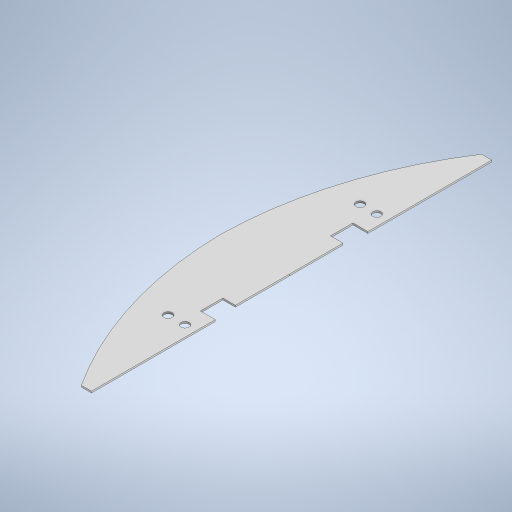
# Autodesk Inventor part: sensor3
Saved by Autodesk Inventor 2023 (Build 270158000, 158)
## iProperties
Created: 2023-08-10
Part Number: sensor3
Material: Genérico
Document SubType Name: Modeling
Designer: azeve
Density: 1 g/cm^3
Appearance: Padrão
Author: azeve
Autodesk Inventor part; units mm, degrees
ref_plane "YZ Plane" through (0, 0, 0) normal (1, 0, 0) x (0, 1, 0)
ref_plane "XZ Plane" through (0, 0, 0) normal (0, 1, 0) x (-1, 0, 0)
ref_plane "XY Plane" through (0, 0, 0) normal (0, 0, 1) x (1, 0, 0)
sketch "Esboço1" plane through (0, 0, 0) normal (0, 1, 0) x (-1, 0, 0)
  line L0 (-21.2717, 119.5968) -> (-21.2717, 45.5844)
  line L1 (-19.833, 32.1612) -> (-19.845, 0)
  line L2 (-19.845, 0) -> (21.2756, 0)
  arc A0 (21.2756, 0) -> (-15.209, 119.5968) centre (-204.3398, -3.4636) ccw
  circle A1 centre (-4.8173, 57.4104) radius 2.5
  circle A2 centre (-14.8591, 57.303) radius 2.5
  arc A3 (-15.209, -119.5968) -> (21.2756, 0) centre (-204.3398, 3.4636) ccw
  line L3 (-21.2717, -119.5968) -> (-21.2717, -45.5845)
  circle A4 centre (-4.8173, -57.4105) radius 2.5
  circle A5 centre (-14.8591, -57.3031) radius 2.5
  line L4 (-19.833, -32.1612) -> (-19.845, 0)
  line L5 (-21.2717, 45.5844) -> (-12.3591, 45.5844)
  line L6 (-12.3591, 45.5844) -> (-12.3591, 32.1612)
  line L7 (-12.3591, 32.1612) -> (-19.833, 32.1612)
  line L8 (-19.833, -32.1612) -> (-12.3591, -32.1612)
  line L9 (-12.3591, -32.1612) -> (-12.3591, -45.5845)
  line L10 (-12.3591, -45.5845) -> (-21.2717, -45.5845)
  line L11 (-21.2717, -119.5968) -> (-15.209, -119.5968)
  line L12 (-21.2717, 119.5968) -> (-15.209, 119.5968)
  point P0 (0, 0)
  dimension "d0" = 5
  dimension "d1" = 5
  constraints: 26 end point, 7 symmetric about line, 6 centre point, 4 horizontal, 4 perpendicular, 4 point on circle, 1 vertical, 3 other
  measures "d0" diameter of A1
  measures "d1" diameter of A2
extrude "Extrusão1" add sketch "Esboço1" along normal blind 1
